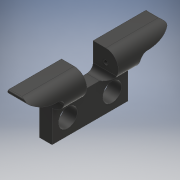
# Autodesk Inventor part: +XPanel_AntennaMount
Saved by Autodesk Inventor 2018 (Build 220112000, 112)
## iProperties
Created: 2018-10-28
Part Number: +XPanel_AntennaMount
Material: Acetal Resin, Black
Document SubType Name: Modeling
Designer: Bradley
Density: 1.425 g/cm^3
Appearance: Smooth - Black
Author: Bradley
Autodesk Inventor part; units mm, degrees
ref_plane "YZ Plane" through (0, 0, 0) normal (1, 0, 0) x (0, 1, 0)
ref_plane "XZ Plane" through (0, 0, 0) normal (0, 1, 0) x (-1, 0, 0)
ref_plane "XY Plane" through (0, 0, 0) normal (0, 0, 1) x (1, 0, 0)
sketch "Sketch1" plane through (0, 0, 0) normal (0, 1, 0) x (-1, 0, 0)
  line L0 (2, -7) -> (2, 2)
  line L1 (2, 2) -> (0, 2)
  arc A0 (0, 2) -> (0, -2) centre (0, 0) ccw
  line L2 (0, -2) -> (0, -7)
  line L3 (0, -7) -> (2, -7)
  circle A1 centre (0, 0) radius 0.35
  dimension "d0" = 5
  dimension "d1" = 2
  dimension "d2" = 2
  dimension "d3" = 0.7
  constraints: 9 end point, 2 centre point, 2 coincident, 2 perpendicular, 2 point on circle, 1 line through centre, 1 parallel, 1 tangent, 1 vertical
  measures "d0" distance of L2.start L2.end
  measures "d1" distance of L2.end L0.start
  measures "d2" radius of A0
  measures "d3" diameter of A1
extrude "Extrusion1" add sketch "Sketch1" along normal mid plane 12
sketch "Sketch2" plane through (0, -6, -7) normal (1, 0, 0) x (0, 0, -1)
  line L0 (0, 12) -> (0, 0) projected
  line L1 (-5, 12) -> (0, 12) projected
  line L2 (-5, 12) -> (-5, 0) projected
  line L3 (0, 0) -> (-5, 0) projected
  circle A0 centre (-2.5, 2.5) radius 2.5 construction
  line L4 (0, 0) -> (-5, 0) construction
  circle A1 centre (-2.5, 9.5) radius 2.5 construction
  line L5 (0, 12) -> (-9, 12) construction
  line L6 (-5, 12) -> (-5, 0) construction
  line L7 (0, 12) -> (0, 0) construction
  point P0 (-7, 6)
  constraints: 6 tangent, 2 centre point, 2 coincident
hole "Hole1" at (0, -3.5, -4.5) at (0, 3.5, -4.5) direction (-1, 0, 0) diameter 3 end through all
sketch "Sketch3" plane through (0, -6, -7) normal (1, 0, 0) x (0, 0, -1)
  circle A0 centre (-2.5, 2.5) radius 1.5 projected
  circle A1 centre (-2.5, 9.5) radius 1.5 projected
  line L0 (0, 12) -> (0, 0) projected
  line L1 (-5, 12) -> (0, 12) projected
  line L2 (-5, 12) -> (-5, 0) projected
  line L3 (0, 0) -> (-5, 0) projected
  line L4 (-9, 3.5) -> (-6, 3.5)
  line L5 (-5, 4.5) -> (-5, 7.5)
  line L6 (-6, 8.5) -> (-9, 8.5)
  line L7 (-9, 8.5) -> (-9, 3.5)
  arc A2 (-6, 3.5) -> (-5, 4.5) centre (-6, 4.5) ccw
  arc A3 (-5, 7.5) -> (-6, 8.5) centre (-6, 7.5) ccw
  line L8 (-9, 0) -> (-9, 12) projected
  point P0 (-7, 6)
  point P1 (-9, 6)
  dimension "d13" = 1
  dimension "d14" = 5
  constraints: 8 end point, 4 point on circle, 4 tangent, 2 centre point, 2 collinear, 2 midpoint, 2 parallel, 1 equal radius, 1 horizontal, 1 perpendicular
  measures "d13" radius of A2
  measures "d14" distance between parallel lines of L4 L6
extrude "Extrusion2" cut sketch "Sketch3" along normal through all both and the other way through all contours L2 A2 L4 L7 L6 A3
sketch "Sketch4" plane through (0, -6, 0) normal (0, -1, 0) x (1, 0, 0)
  circle A0 centre (0, 0) radius 0.35 projected
  line L0 (-2, 2) -> (-2, -7) projected
  line L1 (-2, -7) -> (0, -7) projected
  line L2 (0, -7) -> (0, -2) projected
  arc A1 (0, -2) -> (0, 2) centre (0, 0) ccw projected
  line L3 (0, 2) -> (-2, 2) projected
  arc A2 (0, -2) -> (0, 2) centre (0, 0) ccw projected
  line L4 (0, -7) -> (0, -2) projected
  line L5 (0, -2) -> (-2, -2)
  line L6 (-2, 2) -> (-2, -7) projected
  constraints: 2 end point, 1 perpendicular, 1 point on line
extrude "Extrusion3" add sketch "Sketch4" along normal blind 10 contours L3 A1 L5 L0
sketch "Sketch5" plane through (-2, -6, -7) normal (-1, 0, 0) x (0, 0, 1)
  line L0 (9, 3.5) -> (6, 3.5) projected
  arc A0 (5, 4.5) -> (6, 3.5) centre (6, 4.5) ccw projected
  line L1 (5, 4.5) -> (5, 7.5) projected
  arc A1 (6, 8.5) -> (5, 7.5) centre (6, 7.5) ccw projected
  line L2 (6, 8.5) -> (9, 8.5) projected
  line L3 (9, 8.5) -> (9, 12) projected
  line L4 (0, 12) -> (9, 12) projected
  line L5 (0, 12) -> (0, 0) projected
  line L6 (5, 0) -> (0, 0) projected
  line L7 (5, 0) -> (5, -10) projected
  line L8 (9, -10) -> (5, -10) projected
  line L9 (9, -10) -> (9, 3.5) projected
  circle A2 centre (2.5, 9.5) radius 1.5 projected
  circle A3 centre (2.5, 2.5) radius 1.5 projected
  arc A4 (7.35, -1) -> (6.35, 0) centre (6.35, -1) ccw
  line L10 (9, 3.5) -> (9, -10) projected
  arc A5 (7.35, -1) -> (9, -5.5141) centre (14.35, -1) ccw
  line L11 (5, 4.5) -> (5, 0) projected
  line L12 (5, 0) -> (6.35, 0)
  line L13 (7.35, -10) -> (6.65, -10) construction
  line L14 (6, 3.5) -> (9, 3.5) construction
  line L15 (9, -10) -> (9, 3.5) construction
  line L16 (9, -5.5141) -> (9, -10)
  line L17 (7.35, -10) -> (7.35, 3.5) projected
  arc A6 (8.5426, -4.9082) -> (9, -4.7686) centre (8.75, -4.7686) ccw
  line L18 (9, -5.5141) -> (9, -4.7686)
  point P0 (7, 6)
  dimension "d19" = 7
  dimension "d22" = 0.25
  dimension "d23" = 33.939
  constraints: 7 point on circle, 6 end point, 6 tangent, 3 centre point, 2 collinear, 2 point on line, 1 equal radius, 1 horizontal alignment, 1 perpendicular
  measures "d19" radius of A5
  measures "d22" radius of A6
extrude "Extrusion4" cut sketch "Sketch5" against normal through all contours L9 A5 A6 | L17 L8 L7 L12 A4 | A5 L9 L8 L17
mirror "Mirror1" about plane through (0, 0, 0) normal (0, 1, 0) of "Extrusion3", "Extrusion4"
body "Solid1"
